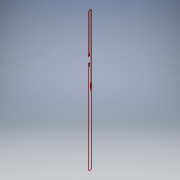
# Autodesk Inventor part: second stage belt 2
Saved by Autodesk Inventor 2017 SP1 (Build 210196100, 196)
## iProperties
Created: 2018-01-21
Part Number: second stage belt 2
Material: Nylon 6/6
Document SubType Name: Modeling
Designer: Ben
Density: 1.13 g/cm^3
Appearance: Light Red
Mass: 35.9399 g
Surface Area: 567.611 cm^2
Volume: 38.645 cm^3
Author: Ben
Autodesk Inventor part; units mm, degrees
ref_plane "YZ Plane" through (0, 0, 0) normal (1, 0, 0) x (0, 1, 0)
ref_plane "XZ Plane" through (0, 0, 0) normal (0, 1, 0) x (-1, 0, 0)
ref_plane "XY Plane" through (0, 0, 0) normal (0, 0, 1) x (1, 0, 0)
sketch "Sketch1" plane through (0, 0, 0) normal (1, 0, 0) x (0, 1, 0)
  line L0 (564.896, 0) -> (251.3795, 0)
  arc A0 (564.896, -19.05) -> (564.896, 0) centre (564.896, -9.525) ccw
  line L1 (564.896, -19.05) -> (21.3158, -19.05)
  arc A1 (-616.204, 0) -> (-616.204, -19.05) centre (-616.204, -9.525) ccw
  line L2 (-616.204, -19.05) -> (-21.3158, -19.05)
  line L3 (21.3158, -23.8125) -> (564.896, -23.8125)
  arc A2 (564.896, -23.8125) -> (564.896, 4.7625) centre (564.896, -9.525) ccw
  line L4 (564.896, 4.7625) -> (251.3795, 4.7625)
  arc A3 (-616.204, 4.7625) -> (-616.204, -23.8125) centre (-616.204, -9.525) ccw
  line L5 (-616.204, -23.8125) -> (-21.3158, -23.8125)
  arc A4 (1.1854, -11.138) -> (-1.1854, -11.138) centre (0, -18.9865) ccw
  arc A5 (21.3158, -19.05) -> (20.3674, -19.1212) centre (21.3158, -25.4) ccw
  line L6 (20.3674, -19.1212) -> (7.6674, -21.0394)
  arc A6 (21.3158, -23.8125) -> (21.0787, -23.8303) centre (21.3158, -25.4) ccw
  line L7 (21.0787, -23.8303) -> (1.1854, -26.835)
  arc A7 (20.3674, -18.8518) -> (21.3158, -18.923) centre (21.3158, -12.573) ccw
  line L8 (21.3158, -18.923) -> (34.0158, -18.923)
  line L9 (20.3674, -18.8518) -> (7.6674, -16.9336)
  line L10 (21.3158, -18.923) -> (21.3158, -19.05) construction
  line L11 (34.0158, -18.923) -> (34.0158, -14.1605)
  line L12 (34.0158, -14.1605) -> (21.3158, -14.1605)
  arc A8 (21.0787, -14.1427) -> (21.3158, -14.1605) centre (21.3158, -12.573) ccw
  line L13 (21.0787, -14.1427) -> (1.1854, -11.138)
  arc A9 (-21.0787, -23.8303) -> (-21.3158, -23.8125) centre (-21.3158, -25.4) ccw
  arc A10 (-20.3674, -19.1212) -> (-21.3158, -19.05) centre (-21.3158, -25.4) ccw
  line L14 (-20.3674, -19.1212) -> (-7.6674, -21.0394)
  arc A11 (-1.1854, -26.835) -> (1.1854, -26.835) centre (0, -18.9865) ccw
  line L15 (-1.1854, -26.835) -> (-21.0787, -23.8303)
  arc A12 (-21.3158, -18.923) -> (-20.3674, -18.8518) centre (-21.3158, -12.573) ccw
  line L16 (-21.3158, -19.05) -> (-21.3158, -18.923) construction
  line L17 (-21.3158, -18.923) -> (-34.0158, -18.923)
  line L18 (-34.0158, -18.923) -> (-34.0158, -14.1605)
  line L19 (-34.0158, -14.1605) -> (-21.3158, -14.1605)
  arc A13 (-21.3158, -14.1605) -> (-21.0787, -14.1427) centre (-21.3158, -12.573) ccw
  line L20 (-21.0787, -14.1427) -> (-1.1854, -11.138)
  line L21 (162.958, 0) -> (-616.204, 0)
  line L22 (162.958, 4.7625) -> (-616.204, 4.7625)
  arc A14 (237.2515, 3.0937) -> (237.2221, -3.1003) centre (236.5375, 0) ccw
  arc A15 (249.9515, 0.1626) -> (251.3795, 0) centre (251.3795, 6.35) ccw
  line L23 (249.9515, 0.1626) -> (237.2515, 3.0937)
  line L24 (251.0225, 4.8032) -> (238.3225, 7.7342)
  arc A16 (238.3225, 7.7342) -> (238.2491, -7.7508) centre (236.5375, 0) ccw
  arc A17 (7.6674, -21.0394) -> (7.6674, -16.9336) centre (0, -18.9865) ccw
  line L25 (-7.6674, -16.9336) -> (-20.3674, -18.8518)
  arc A18 (1.1854, -11.138) -> (-1.1854, -11.138) centre (0, -18.9865) ccw
  arc A19 (-7.6674, -16.9336) -> (-7.6674, -21.0394) centre (0, -18.9865) ccw
  arc A20 (-1.1854, -26.835) -> (1.1854, -26.835) centre (0, -18.9865) ccw
  circle A21 centre (0, -18.9865) radius 3.175
  arc A22 (251.0225, 4.8032) -> (251.3795, 4.7625) centre (251.3795, 6.35) ccw
  arc A23 (251.3795, -0.127) -> (250.0102, -0.2764) centre (251.3795, -6.477) ccw
  arc A24 (251.3795, -4.8895) -> (251.0372, -4.9268) centre (251.3795, -6.477) ccw
  line L26 (251.3795, -0.127) -> (264.0795, -0.127)
  line L27 (264.0795, -0.127) -> (264.0795, -4.8895)
  line L28 (264.0795, -4.8895) -> (251.3795, -4.8895)
  line L29 (250.0102, -0.2764) -> (237.2221, -3.1003)
  line L30 (238.2491, -7.7508) -> (251.0372, -4.9268)
  line L31 (251.3795, 0) -> (251.3795, -0.127) construction
  arc A25 (177.1154, -3.1003) -> (177.086, 3.0937) centre (177.8, 0) ccw
  arc A26 (176.0884, -7.7508) -> (176.015, 7.7342) centre (177.8, 0) ccw
  arc A27 (162.958, 0) -> (164.386, 0.1626) centre (162.958, 6.35) ccw
  arc A28 (162.958, 4.7625) -> (163.315, 4.8032) centre (162.958, 6.35) ccw
  line L32 (177.086, 3.0937) -> (164.386, 0.1626)
  line L33 (176.015, 7.7342) -> (163.315, 4.8032)
  arc A29 (164.3273, -0.2764) -> (162.958, -0.127) centre (162.958, -6.477) ccw
  arc A30 (163.3003, -4.9268) -> (162.958, -4.8895) centre (162.958, -6.477) ccw
  line L34 (162.958, -0.127) -> (150.258, -0.127)
  line L35 (150.258, -0.127) -> (150.258, -4.8895)
  line L36 (150.258, -4.8895) -> (162.958, -4.8895)
  line L37 (177.1154, -3.1003) -> (164.3273, -0.2764)
  line L38 (176.0884, -7.7508) -> (163.3003, -4.9268)
  line L39 (162.958, -0.127) -> (162.958, 0) construction
  line L40 (0, 0) -> (0, -18.9865) construction
  dimension "d1" = 9.525
  dimension "d5" = 4.7625
  dimension "d7" = 6.35
  dimension "d9" = 12.7
  dimension "d10" = 0.127
  dimension "d11" = 6.35
  dimension "d13" = 0.127
  dimension "d14" = 12.7
  dimension "d15" = 1181.1
  dimension "d20" = 6.35
  dimension "d22" = 12.7
  dimension "d23" = 12.7
  dimension "d24" = 0.127
  dimension "d25" = 12.7
  dimension "d27" = 58.7375
  dimension "d30" = 177.8
  dimension "d31" = 616.204
  dimension "d32" = 9.525
  constraints: 82 end point, 61 point on circle, 56 tangent, 31 centre point, 12 coincident, 9 horizontal, 9 parallel, 8 equal radius, 7 equal length, 6 perpendicular, 5 vertical, 3 point on line, 2 collinear, 1 concentric, 1 line through centre, 2 other
  measures "d1" radius of A0
  measures "d5" distance between parallel lines of L4 L0
  measures "d7" radius of A5
  measures "d9" distance of L8.start L8.end
  measures "d10" distance between parallel lines of L8 L1
  measures "d11" radius of A10
  measures "d13" distance of L2.end L16.end
  measures "d14" distance of L16.end L17.end
  measures "d15" distance of A1.centre A0.centre
  measures "d20" diameter of A21
  measures "d22" horizontal distance of L9.start L9.end
  measures "d23" horizontal distance of L23.start L23.end
  measures "d24" distance between parallel lines of L26 L0
  measures "d25" distance of L27.end L28.end
  measures "d27" distance of A14.centre A25.centre
  measures "d30" distance from line of L40 A25.centre
  measures "d31" distance from line of A1.centre L40
  measures "d32" radius of A1
extrude "Extrusion1" add sketch "Sketch1" along normal mid plane 4.7625
fillet "Fillet1" radius 1.5875 68 edges at (2.3813, -226.623, 0) (2.3813, 163.6766, 0.0408) (2.3813, 170.736, 1.6282) (2.3813, 180.975, 0.0151) (2.3813, 170.7213, -1.6883) (2.3813, 163.6467, -0.1645) (2.3813, 156.608, -0.127) (2.3813, -318.7599, -19.05) (2.3813, -20.8403, -19.0678) (2.3813, -14.0174, -20.0803) (2.3813, -625.729, -9.525) (2.3813, -318.7599, -23.8125) (2.3813, -21.1969, -23.817) (2.3813, -11.1321, -25.3326) (2.3813, 0, -26.924) (2.3813, 11.1321, -25.3326) (2.3813, 21.1969, -23.817) (2.3813, 293.1059, -23.8125) (2.3813, 579.1835, -9.525) (2.3813, 408.1377, 4.7625) (2.3813, 251.1998, 4.7727) (2.3813, 244.6725, 6.2687) (2.3813, 228.6001, 0.0376) (2.3813, 244.6431, -6.3388) (2.3813, 251.2073, -4.8989) (2.3813, 257.7295, -4.8895) (2.3813, -226.623, 4.7625) (2.3813, 163.1377, 4.7727) (2.3813, 169.665, 6.2687) (2.3813, 185.7374, 0.0376) (2.3813, 169.6944, -6.3388) (2.3813, 163.1302, -4.8989) (2.3813, 156.608, -4.8895) (2.3813, -630.4915, -9.525) (-2.3813, -226.623, 4.7625) (-2.3813, 163.1377, 4.7727) (-2.3813, 169.665, 6.2687) (-2.3813, 185.7374, 0.0376) (-2.3813, 169.6944, -6.3388) (-2.3813, 163.1302, -4.8989) (-2.3813, 156.608, -4.8895) (-2.3813, -318.7599, -23.8125) (-2.3813, -21.1969, -23.817) (-2.3813, -11.1321, -25.3326) (-2.3813, 0, -26.924) (-2.3813, 11.1321, -25.3326) (-2.3813, 21.1969, -23.817) (-2.3813, 293.1059, -23.8125) (-2.3813, 579.1835, -9.525) (-2.3813, 408.1377, 4.7625) (-2.3813, 251.1998, 4.7727) (-2.3813, 244.6725, 6.2687) (-2.3813, 228.6001, 0.0376) (-2.3813, 244.6431, -6.3388) (-2.3813, 251.2073, -4.8989) (-2.3813, 257.7295, -4.8895) (-2.3813, -630.4915, -9.525) (-2.3813, -318.7599, -19.05) (-2.3813, -20.8403, -19.0678) (-2.3813, -14.0174, -20.0803) (-2.3813, -226.623, 0) (-2.3813, 163.6766, 0.0408) (-2.3813, 170.736, 1.6282) (-2.3813, 180.975, 0.0151) (-2.3813, 170.7213, -1.6883) (-2.3813, 163.6467, -0.1645) (-2.3813, 156.608, -0.127) (-2.3813, -625.729, -9.525)
body "Solid1"
